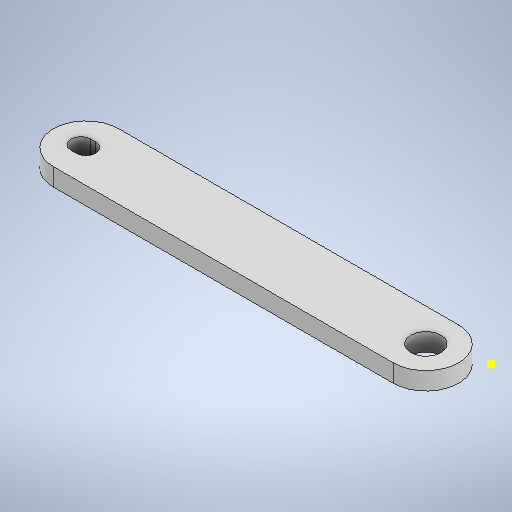
# Autodesk Inventor part: crankRod1
Saved by Autodesk Inventor 2025.2 (Build 292293000, 293)
## iProperties
Created: 2025-03-20
Part Number: crankRod1
Material: Generic
Document SubType Name: Modeling
Designer: patrickandersen
Density: 1 g/cm^3
Appearance: Default
Author: patrickandersen
Autodesk Inventor part; units mm, degrees
ref_plane "YZ Plane" through (0, 0, 0) normal (1, 0, 0) x (0, 1, 0)
ref_plane "XZ Plane" through (0, 0, 0) normal (0, 1, 0) x (-1, 0, 0)
ref_plane "XY Plane" through (0, 0, 0) normal (0, 0, 1) x (1, 0, 0)
sketch "Sketch1" plane through (0, 0, 0) normal (0, 1, 0) x (-1, 0, 0)
  line L0 (0, 0) -> (114.5, 0)
  line L1 (114.5, 0) -> (114.5, 18.5)
  line L2 (114.5, 18.5) -> (0, 18.5)
  line L3 (0, 18.5) -> (0, 0)
  circle A0 centre (105.25, 9.25) radius 2.75
  circle A1 centre (9.25, 9.25) radius 4.25
  dimension "d12" = 5.5
  dimension "d44" = 8.5
  dimension "d52" = 96
  dimension "d57" = 9.25
  dimension "d58" = 9.25
  dimension "d59" = 9.25
  dimension "d60" = 9.25
  constraints: 8 end point, 2 centre point, 2 parallel, 1 horizontal, 1 perpendicular
  measures "d12" diameter of A0
  measures "d44" diameter of A1
  measures "d52" distance of A1.centre A0.centre
  measures "d57" distance from line of L3 A1.centre
  measures "d58" distance from line of A0.centre L1
  measures "d59" distance from line of L2 A1.centre
  measures "d60" distance from line of L0 A1.centre
extrude "Extrusion3" add sketch "Sketch1" along normal blind 5
fillet "Fillet3" radius 9.25 1 edges at (-114.5, 2.5, 0)
fillet "Fillet4" radius 9.25 3 edges at (-114.5, 2.5, 18.5) (0, 2.5, 18.5) (0, 2.5, 0)
sketch "Sketch2" plane through (0, 0, 0) normal (0, -1, 0) x (1, 0, 0)
  point P0 (0, 0)
sketch "Sketch3" plane through (0, 5, 0) normal (0, 1, 0) x (1, 0, 0)
  circle A0 centre (-105.25, -9.25) radius 2.75 projected
  circle A1 centre (-106.75, -9.25) radius 2.75
  line L0 (-106.75, -6.5) -> (-105.25, -6.5)
  line L1 (-105.25, -12) -> (-106.75, -12)
  line L2 (-106.75, -6.5) -> (-105.25, -6.5)
  line L3 (-106.75, -12) -> (-105.25, -12)
  point P0 (0, 0)
  dimension "d62" = 5.5
  dimension "d64" = 1.5
  constraints: 8 end point, 5 tangent, 4 point on circle, 3 equal length, 1 centre point
  measures "d62" diameter of A1
  measures "d64" distance of A0.centre A1.centre
extrude "Extrusion4" cut sketch "Sketch3" against normal blind 10 contours A0 A1 L0 | L1 A1 A0 | A0 A1 picked at (-108.9803, -9.1424)
body "Solid2"
